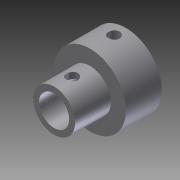
# Autodesk Inventor part: sprocket hub adaptor
Saved by Autodesk Inventor 2012 (Build 160160000, 160)
## iProperties
Created: 2013-07-25
Part Number: sprocket hub adaptor
Material: Default
Document SubType Name: Modeling
Designer: Bryce
Density: 1 g/cm^3
Author: Bryce
Autodesk Inventor part; units mm, degrees
ref_plane "YZ Plane" through (0, 0, 0) normal (1, 0, 0) x (0, 1, 0)
ref_plane "XZ Plane" through (0, 0, 0) normal (0, 1, 0) x (-1, 0, 0)
ref_plane "XY Plane" through (0, 0, 0) normal (0, 0, 1) x (1, 0, 0)
sketch "Sketch1" plane through (0, 0, 0) normal (0, 0, 1) x (1, 0, 0)
  circle A0 centre (0, 0) radius 7.1437
  circle A1 centre (0, 0) radius 9.525
  circle A2 centre (0, 0) radius 4
  circle A3 centre (0, 0) radius 5.5563
  dimension "d0" = 14.2875
  dimension "d1" = 19.05
  dimension "d2" = 8
  dimension "d3" = 11.1125
  constraints: 4 centre point, 4 coincident
  measures "d0" diameter of A0
  measures "d1" diameter of A1
  measures "d2" diameter of A2
  measures "d3" diameter of A3
extrude "Extrusion1" add sketch "Sketch1" along normal blind 3.175 contours A0 | A1 | A3
extrude "Extrusion2" add sketch "Sketch1" along normal blind 12.7 contours A3
extrude "Extrusion3" add sketch "Sketch1" against normal blind 6.35 contours A1
sketch "Sketch2" plane through (0, 0, 0) normal (0, 1, 0) x (-1, 0, 0)
  circle A0 centre (0, 7.9375) radius 1.5
  circle A1 centre (0, -3.175) radius 1.5
  line L0 (-7.1437, 0) -> (7.1437, 0) projected
  line L1 (-4, 12.7) -> (4, 12.7) projected
  point P0 (0, 0)
  point P1 (0, 0)
  dimension "d10" = 3
  dimension "d11" = 3.175
  dimension "d12" = 4.7625
  constraints: 2 centre point, 2 vertical alignment, 1 equal radius, 1 midpoint
  measures "d10" diameter of A0
  measures "d11" distance from line of A1.centre L0
  measures "d12" distance from line of L1 A0.centre
extrude "Extrusion4" cut sketch "Sketch2" along normal through all
body "Solid1"
